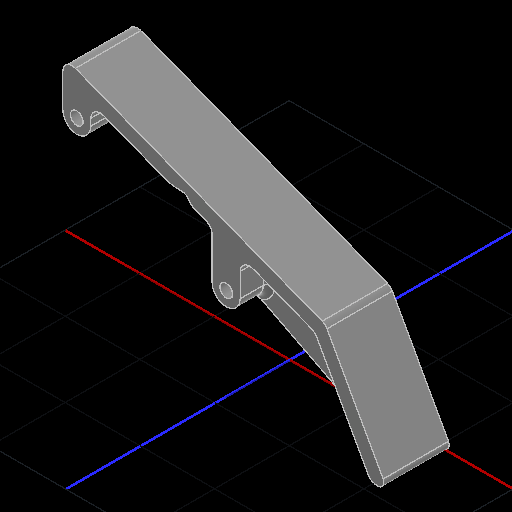
# Autodesk Inventor part: funnel
Saved by Autodesk Inventor 2025.2 (Build 292293000, 293)
## iProperties
Created: 2025-11-17
Part Number: funnel
Material: white pla
Document SubType Name: Modeling
Designer: cloudy
Density: 1 g/cm^3
Appearance: Smooth - Dark Gray
Author: cloudy
Autodesk Inventor part; units mm, degrees
ref_plane "YZ Plane" through (0, 0, 0) normal (1, 0, 0) x (0, 1, 0)
ref_plane "XZ Plane" through (0, 0, 0) normal (0, 1, 0) x (-1, 0, 0)
ref_plane "XY Plane" through (0, 0, 0) normal (0, 0, 1) x (1, 0, 0)
sketch "Sketch1" plane through (0, 0, 0) normal (0, 0, 1) x (1, 0, 0)
  circle A0 centre (-50.024865, 184.15) radius 2.1844
  circle A1 centre (0.775135, 158.75) radius 2.1844
  line L0 (-38.265507, 111.59275) -> (-11.417832, 111.59275) construction
  line L1 (-11.417832, 111.59275) -> (-11.417832, 180.50725)
  line L2 (-11.417832, 180.50725) -> (-38.265507, 180.50725)
  line L3 (-38.265507, 180.50725) -> (-38.265507, 111.59275) construction
  line L4 (-38.265507, 111.59275) -> (-11.417832, 180.50725) construction
  line L5 (-11.417832, 111.59275) -> (-38.265507, 180.50725) construction
  line L6 (-59.666221, -167.868068) -> (-59.666221, 213.131932) construction
  circle A2 centre (-50.024865, 184.15) radius 4.7625
  line L7 (-45.262365, 191.139086) -> (-3.987365, 175.141704)
  circle A3 centre (0.775135, 158.75) radius 4.7625
  line L8 (-3.987365, 158.75) -> (-3.987365, 175.141704)
  line L9 (34.497486, 165.67394) -> (-54.787365, 200.279)
  line L10 (-45.262365, 184.15) -> (-45.262365, 191.139086)
  line L11 (-54.787365, 184.15) -> (-54.787365, 200.279)
  line L12 (-54.787365, 200.279) -> (14.748968, 173.328079)
  line L13 (5.537635, 158.75) -> (5.537635, 171.45)
  line L14 (34.497486, 165.67394) -> (55.771538, 127)
  line L15 (55.771538, 127) -> (49.973666, 127)
  line L16 (49.973666, 127) -> (30.937635, 161.605457)
  line L17 (5.537635, 171.45) -> (30.937635, 161.605457)
  line L18 (107.785335, 127) -> (46.317335, 127)
  point P0 (0, 0)
  point P1 (-24.84167, 146.05)
  point P2 (-17.831062, 180.50725)
  point P3 (-11.417832, 178.021607)
  dimension "d1" = 381
  dimension "d2" = 9.525
  dimension "d4" = 9.525
  dimension "d5" = 5.08
  dimension "d6" = 12.7
  dimension "d7" = 16.129
  dimension "d8" = 140
  dimension "d9" = 5.08
  dimension "d10" = 25.4
  constraints: 36 end point, 6 vertical, 4 parallel, 4 point on circle, 4 tangent, 3 collinear, 3 horizontal, 2 centre point, 2 coincident, 2 midpoint, 1 perpendicular, 1 other
  measures "d1" distance of L6.start L6.end
  measures "d2" diameter of A2
  measures "d4" diameter of A3
  measures "d5" distance between parallel lines of L12 L7
  measures "d6" distance of L13.start L13.end
  measures "d7" distance of L9.end L11.start
  measures "d8" angle of L16 L17
  measures "d9" distance between parallel lines of L14 L16
  measures "d10" distance from line of L13 L16.end
extrude "Extrusion1" add sketch "Sketch1" along normal blind 22.225 contours L1 L2 L7 L10 A2 L11 L9 L14 L15 L16 L17 L13 A3 L8 | A3 | A2
fillet "Fillet1" radius 3.175 7 edges at (-54.7874, 200.279, 11.1125) (-45.2624, 191.1391, 11.1125) (-3.9874, 175.1417, 11.1125) (5.5376, 171.45, 11.1125) (30.9376, 161.6055, 11.1125) (34.4975, 165.6739, 11.1125) (49.9737, 127, 11.1125)
fillet "Fillet2" radius 2 1 edges at (55.7715, 127, 11.1125)
ref_plane "Work Plane1" through (0, 0, 11.1125) normal (0, 0, 1) x (1, 0, 0)
sketch "Sketch2" plane through (0, 0, 11.1125) normal (0, 0, 1) x (1, 0, 0)
  line L0 (5.537635, 158.75) -> (5.537635, 166.8143) construction
  line L1 (-1.397209, 154.511802) -> (49.068925, 128.644721)
  line L2 (31.494611, 160.592935) -> (49.068925, 128.644721) construction
  arc A0 (-3.987365, 158.75) -> (5.537635, 158.75) centre (0.775135, 158.75) ccw
  point P0 (0, 0)
  constraints: 2 end point, 1 point on circle, 1 tangent
extrude "Rib1" add sketch "Sketch2" along normal mid plane 2.54 rib yes fills toward (23.858665, 141.622757) open curves L1
fillet "Fillet3" radius 2 10 edges at (6.9185, 169.4338, 12.3825) (19.8601, 165.8989, 12.3825) (30.8035, 161.4521, 12.3825) (40.2818, 144.6188, 12.3825) (5.5376, 162.7822, 12.3825) (6.9185, 169.4338, 9.8425) (19.8601, 165.8989, 9.8425) (30.8035, 161.4521, 9.8425) (40.2818, 144.6188, 9.8425) (5.5376, 162.7822, 9.8425)
fillet "Fillet4" radius 12.7 1 edges at (-17.8311, 180.5072, 11.1125)
fillet "Fillet5" radius 3 2 edges at (-11.4178, 180.5072, 11.1125) (-11.4178, 178.0216, 11.1125)
body "Solid1"
